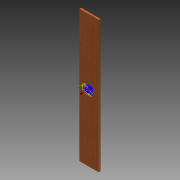
# Autodesk Inventor part: placa spate
Saved by Autodesk Inventor 2015 SP1 (Build 190203100, 203)
## iProperties
Created: 2015-04-26
Part Number: placa spate
Material: Wood (Cherry)
Document SubType Name: Modeling
Designer: ubik
Density: 0.63 g/cm^3
Appearance: Cherry - Natural Low Gloss
Author: ubik
Autodesk Inventor part; units mm, degrees
ref_plane "YZ Plane" through (0, 0, 0) normal (1, 0, 0) x (0, 1, 0)
ref_plane "XZ Plane" through (0, 0, 0) normal (0, 1, 0) x (-1, 0, 0)
ref_plane "XY Plane" through (0, 0, 0) normal (0, 0, 1) x (1, 0, 0)
sketch "Sketch1" plane through (0, 0, 0) normal (0, 0, 1) x (1, 0, 0)
  line L0 (0, 0) -> (-69.8501, 0)
  line L1 (-69.8501, 0) -> (-69.8501, 600.075)
  line L2 (-69.8501, 600.075) -> (0, 600.075)
  line L3 (0, 600.075) -> (0, 0)
  line L4 (-56.1086, 321.0499) -> (-23.8915, 321.0499) projected
  line L5 (-23.8915, 321.0499) -> (-18.9501, 316.1085) projected
  line L6 (-18.9501, 316.1085) -> (-18.9501, 283.8914) projected
  line L7 (-61.0501, 316.1085) -> (-56.1086, 321.0499) projected
  line L8 (-61.0501, 283.8914) -> (-61.0501, 316.1085) projected
  line L9 (-56.1086, 278.9499) -> (-61.0501, 283.8914) projected
  line L10 (-23.8915, 278.9499) -> (-56.1086, 278.9499) projected
  line L11 (-18.9501, 283.8914) -> (-23.8915, 278.9499) projected
  dimension "d2" = 8.8
  dimension "d3" = 18.9501
  constraints: 8 end point, 2 parallel, 1 horizontal, 1 perpendicular
  measures "d2" distance between parallel lines of L1 L8
  measures "d3" distance between parallel lines of L3 L6
extrude "Extrusion1" add sketch "Sketch1" along normal blind 8
sketch "Sketch2" plane through (-69.8501, 0, 0) normal (-1, 0, 0) x (0, 0, 1)
  line L0 (0, 0) -> (0, 600.075) projected
  line L1 (0, 0) -> (8, 0) projected
  line L2 (8, 600.075) -> (8, 0) projected
  line L3 (0, 600.075) -> (8, 600.075) projected
  point P0 (0, 0)
extrude "Extrusion2" add sketch "Sketch2" along normal blind 9
sketch "Sketch3" plane through (0, 0, 0) normal (1, 0, 0) x (0, 0, -1)
  line L0 (0, 600.075) -> (0, 0) projected
  line L1 (0, 600.075) -> (-8, 600.075) projected
  line L2 (-8, 0) -> (-8, 600.075) projected
  line L3 (0, 0) -> (-8, 0) projected
extrude "Extrusion3" add sketch "Sketch3" along normal blind 9
body "Solid1"
